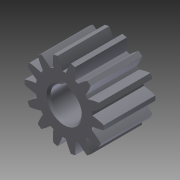
# Autodesk Inventor part: am-0741
Saved by Autodesk Inventor 2012 (Build 160160000, 160)
## iProperties
Category: Drive Base Kit
Company: Autodesk Inc.
Created: 2011-12-23
Part Number: am-0741
Material: Default
Document SubType Name: Modeling
Designer: Autodesk Inc.
Density: 1 g/cm^3
Catalog Web Link: http://www.andymark.com/product-p/am-0741.htm
Description: 12 tooth CIM gear
Vendor: AndyMark
Author: Autodesk Inc.
Autodesk Inventor part; units mm, degrees
ref_plane "YZ Plane" through (0, 0, 0) normal (1, 0, 0) x (0, 1, 0)
ref_plane "XZ Plane" through (0, 0, 0) normal (0, 1, 0) x (-1, 0, 0)
ref_plane "XY Plane" through (0, 0, 0) normal (0, 0, 1) x (1, 0, 0)
sketch "Sketch1" plane through (0, 0, 0) normal (0, 0, 1) x (1, 0, 0)
  arc A0 (-3.1269, -1.4516) -> (-2.9447, -0.6532) centre (-10.144, 0.57) ccw
  arc A1 (-2.9447, -0.6532) -> (0, 0) centre (-4.7545, 14.4689) ccw
  line L0 (0, 0) -> (0, 1.1399)
  arc A2 (0, 1.1399) -> (-2.9447, 1.7932) centre (-4.7545, -13.329) ccw
  arc A3 (-2.9447, 1.7932) -> (-3.1269, 2.5916) centre (-10.144, 0.57) ccw
  arc A4 (-3.1269, 2.5916) -> (-0.7573, 4.4578) centre (-11.3188, 15.4309) ccw
  line L1 (-0.7573, 4.4578) -> (-1.2519, 5.4848)
  arc A5 (-1.2519, 5.4848) -> (-4.1884, 4.7957) centre (0.7423, -9.6141) ccw
  arc A6 (-4.1884, 4.7957) -> (-4.699, 5.436) centre (-10.144, 0.57) ccw
  arc A7 (-4.699, 5.436) -> (-3.3737, 8.1455) centre (-17.6504, 13.4495) ccw
  line L2 (-3.3737, 8.1455) -> (-4.265, 8.8563)
  arc A8 (-4.265, 8.8563) -> (-6.6117, 6.9613) centre (4.0829, -3.8822) ccw
  arc A9 (-6.6117, 6.9613) -> (-7.3495, 7.3166) centre (-10.144, 0.57) ccw
  arc A10 (-7.3495, 7.3166) -> (-7.3311, 10.3328) centre (-22.4952, 8.9171) ccw
  line L3 (-7.3311, 10.3328) -> (-8.4425, 10.5865)
  arc A11 (-8.4425, 10.5865) -> (-9.7346, 7.861) centre (4.6057, 2.7315) ccw
  arc A12 (-9.7346, 7.861) -> (-10.5535, 7.861) centre (-10.144, 0.57) ccw
  arc A13 (-10.5535, 7.861) -> (-11.8456, 10.5865) centre (-24.8938, 2.7315) ccw
  line L4 (-11.8456, 10.5865) -> (-12.957, 10.3328)
  arc A14 (-12.957, 10.3328) -> (-12.9386, 7.3166) centre (2.2072, 8.9171) ccw
  arc A15 (-12.9386, 7.3166) -> (-13.6764, 6.9613) centre (-10.144, 0.57) ccw
  arc A16 (-13.6764, 6.9613) -> (-16.0231, 8.8563) centre (-24.371, -3.8822) ccw
  line L5 (-16.0231, 8.8563) -> (-16.9143, 8.1455)
  arc A17 (-16.9143, 8.1455) -> (-15.5891, 5.436) centre (-2.6377, 13.4495) ccw
  arc A18 (-15.5891, 5.436) -> (-16.0997, 4.7957) centre (-10.144, 0.57) ccw
  arc A19 (-16.0997, 4.7957) -> (-19.0362, 5.4848) centre (-21.0303, -9.6141) ccw
  line L6 (-19.0362, 5.4848) -> (-19.5308, 4.4578)
  arc A20 (-19.5308, 4.4578) -> (-17.1611, 2.5916) centre (-8.9693, 15.4309) ccw
  arc A21 (-17.1611, 2.5916) -> (-17.3433, 1.7932) centre (-10.144, 0.57) ccw
  arc A22 (-17.3433, 1.7932) -> (-20.288, 1.1399) centre (-15.5335, -13.329) ccw
  line L7 (-20.288, 1.1399) -> (-20.288, 0)
  arc A23 (-20.288, 0) -> (-17.3433, -0.6532) centre (-15.5335, 14.4689) ccw
  arc A24 (-17.3433, -0.6532) -> (-17.1611, -1.4516) centre (-10.144, 0.57) ccw
  arc A25 (-17.1611, -1.4516) -> (-19.5308, -3.3178) centre (-8.9693, -14.291) ccw
  line L8 (-19.5308, -3.3178) -> (-19.0362, -4.3449)
  arc A26 (-19.0362, -4.3449) -> (-16.0997, -3.6558) centre (-21.0303, 10.7541) ccw
  arc A27 (-16.0997, -3.6558) -> (-15.5891, -4.296) centre (-10.144, 0.57) ccw
  arc A28 (-15.5891, -4.296) -> (-16.9143, -7.0056) centre (-2.6377, -12.3096) ccw
  line L9 (-16.9143, -7.0056) -> (-16.0231, -7.7163)
  arc A29 (-16.0231, -7.7163) -> (-13.6764, -5.8213) centre (-24.371, 5.0222) ccw
  arc A30 (-13.6764, -5.8213) -> (-12.9386, -6.1767) centre (-10.144, 0.57) ccw
  arc A31 (-12.9386, -6.1767) -> (-12.957, -9.1929) centre (2.2072, -7.7772) ccw
  line L10 (-12.957, -9.1929) -> (-11.8456, -9.4465)
  arc A32 (-11.8456, -9.4465) -> (-10.5535, -6.721) centre (-24.8938, -1.5916) ccw
  arc A33 (-10.5535, -6.721) -> (-9.7346, -6.721) centre (-10.144, 0.57) ccw
  arc A34 (-9.7346, -6.721) -> (-8.4425, -9.4465) centre (4.6057, -1.5916) ccw
  line L11 (-8.4425, -9.4465) -> (-7.3311, -9.1929)
  arc A35 (-7.3311, -9.1929) -> (-7.3495, -6.1767) centre (-22.4952, -7.7772) ccw
  arc A36 (-7.3495, -6.1767) -> (-6.6117, -5.8213) centre (-10.144, 0.57) ccw
  arc A37 (-6.6117, -5.8213) -> (-4.265, -7.7163) centre (4.0829, 5.0222) ccw
  line L12 (-4.265, -7.7163) -> (-3.3737, -7.0056)
  arc A38 (-3.3737, -7.0056) -> (-4.699, -4.296) centre (-17.6504, -12.3096) ccw
  arc A39 (-4.699, -4.296) -> (-4.1884, -3.6558) centre (-10.144, 0.57) ccw
  arc A40 (-4.1884, -3.6558) -> (-1.2519, -4.3449) centre (0.7423, 10.7541) ccw
  line L13 (-1.2519, -4.3449) -> (-0.7573, -3.3178)
  arc A41 (-0.7573, -3.3178) -> (-3.1269, -1.4516) centre (-11.3188, -14.291) ccw
  line L14 (-9.144, 5.57) -> (-11.144, 5.57)
  line L15 (-9.144, 4.443) -> (-9.144, 5.57)
  arc A42 (-11.144, 4.443) -> (-9.144, 4.443) centre (-10.144, 0.57) ccw
  line L16 (-11.144, 5.57) -> (-11.144, 4.443)
  constraints: 86 point on circle, 43 centre point, 34 end point
extrude "Extrusion1" add sketch "Sketch1" against normal blind 13.208
chamfer "Chamfer1" distance 0.508 angle 45 2 edges at (-10.144, -3.43, 0) (-10.144, -3.43, -13.208)
body "Solid1"
